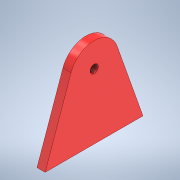
# Autodesk Inventor part: Roller Frame
Saved by Autodesk Inventor 2022.4 (Build 264492000, 492)
## iProperties
Created: 2024-02-15
Part Number: Roller Frame
Material: Generic
Document SubType Name: Modeling
Designer: t60147996
Density: 1 g/cm^3
Appearance: Light Red
Author: t60147996
Autodesk Inventor part; units mm, degrees
ref_plane "YZ Plane" through (0, 0, 0) normal (1, 0, 0) x (0, 1, 0)
ref_plane "XZ Plane" through (0, 0, 0) normal (0, 1, 0) x (-1, 0, 0)
ref_plane "XY Plane" through (0, 0, 0) normal (0, 0, 1) x (1, 0, 0)
sketch "Sketch1" plane through (0, 0, 0) normal (1, 0, 0) x (0, 1, 0)
  line L0 (0, 80.1594) -> (0, -72.2406)
  circle A0 centre (101.6, 3.9594) radius 38.1
  line L1 (0, -72.2406) -> (114.2631, -31.9747)
  line L2 (0, 80.1594) -> (114.2631, 39.8934)
  point P0 (0, 0)
  dimension "d0" = 152.4
  dimension "d1" = 76.2
  dimension "d2" = 101.6
  constraints: 6 end point, 2 point on circle, 2 tangent, 1 centre point, 1 vertical
  measures "d0" distance of L0.start L0.end
  measures "d1" diameter of A0
  measures "d2" distance from line of L0 A0.centre
extrude "Extrusion1" add sketch "Sketch1" along normal blind 12.7
sketch "Sketch2" plane through (12.7, 0, 0) normal (1, 0, 0) x (0, 0, -1)
  arc A0 (31.9747, 114.2631) -> (-39.8934, 114.2631) centre (-3.9594, 101.6) ccw projected
  point P0 (0, 0)
  constraints: 1 coincident
hole "Hole1" at (12.7, 101.6, 3.9594) direction (-1, 0, 0) diameter 12.7 end through all
body "Solid1"
